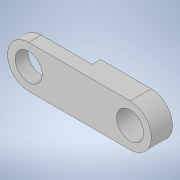
# Autodesk Inventor part: Abzugstange
Saved by Autodesk Inventor 2021 (Build 250183000, 183)
## iProperties
Created: 2021-03-08
Part Number: Abzugstange
Material: Generic
Document SubType Name: Modeling
Designer: Lukas
Density: 1 g/cm^3
Appearance: Default
Author: Lukas
Autodesk Inventor part; units mm, degrees
ref_plane "YZ Plane" through (0, 0, 0) normal (1, 0, 0) x (0, 1, 0)
ref_plane "XZ Plane" through (0, 0, 0) normal (0, 1, 0) x (-1, 0, 0)
ref_plane "XY Plane" through (0, 0, 0) normal (0, 0, 1) x (1, 0, 0)
sketch "Sketch1" plane through (0, 0, 0) normal (0, 0, 1) x (1, 0, 0)
  line L0 (-6, 0) -> (6, 0) construction
  line L1 (-6, -2.5) -> (6, -2.5)
  line L2 (6, 2.5) -> (-6, 2.5)
  arc A0 (-6, 2.5) -> (-6, -2.5) centre (-6, 0) ccw
  arc A1 (6, -2.5) -> (6, 2.5) centre (6, 0) ccw
  circle A2 centre (-6, 0) radius 1.6
  circle A3 centre (6, 0) radius 1.6
  point P0 (0, 0)
  point P1 (0, 0)
  dimension "d56" = 3.2
  dimension "d57" = 12
  dimension "d58" = 5
  constraints: 8 end point, 4 centre point, 4 point on circle, 4 tangent, 3 coincident, 1 equal radius, 1 horizontal, 1 midpoint, 1 parallel
  measures "d56" diameter of A3
  measures "d57" distance of L0.start L0.end
  measures "d58" distance between parallel lines of L1 L2
extrude "Extrusion1" add sketch "Sketch1" along normal blind 2.5
sketch "Sketch5" plane through (-6, 2.5, 0) normal (0, 1, 0) x (1, 0, 0)
  line L0 (-9, 2) -> (6, 2)
  line L1 (6, 2) -> (6, -1)
  line L2 (6, -1) -> (-9, -1)
  line L3 (-9, -1) -> (-9, 2)
  line L4 (12, 0) -> (0, 0) projected
  point P0 (6, 0)
  point P1 (6, 0)
  dimension "d60" = 1
  dimension "d61" = 3
  dimension "d62" = 15
  constraints: 8 end point, 2 parallel, 1 horizontal, 1 midpoint, 1 perpendicular, 1 point on line
  measures "d60" distance from line of point (6, 0) L2
  measures "d61" distance of L2.end L0.start
  measures "d62" distance of L0.start L0.end
extrude "Extrusion5" cut sketch "Sketch5" against normal through all
body "Solid1"
